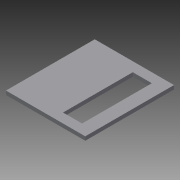
# Autodesk Inventor part: Step Down Regulator Adaptor
Saved by Autodesk Inventor 2015 (Build 190159000, 159)
## iProperties
Created: 2017-12-31
Part Number: Step Down Regulator Adaptor
Material: Generic
Document SubType Name: Modeling
Designer: Toby
Density: 1 g/cm^3
Appearance: Default
Author: Toby
Autodesk Inventor part; units mm, degrees
ref_plane "YZ Plane" through (0, 0, 0) normal (1, 0, 0) x (0, 1, 0)
ref_plane "XZ Plane" through (0, 0, 0) normal (0, 1, 0) x (-1, 0, 0)
ref_plane "XY Plane" through (0, 0, 0) normal (0, 0, 1) x (1, 0, 0)
sketch "Sketch1" plane through (0, 0, 0) normal (0, 0, 1) x (1, 0, 0)
  line L0 (-18.7121, 1.0985) -> (6.2879, 1.0985)
  line L1 (6.2879, 1.0985) -> (6.2879, -26.9015)
  line L2 (6.2879, -26.9015) -> (-18.7121, -26.9015)
  line L3 (-18.7121, -26.9015) -> (-18.7121, 1.0985)
  point P0 (0, 0)
  dimension "d0" = 25
  dimension "d1" = 28
  constraints: 8 end point, 2 parallel, 1 horizontal, 1 perpendicular
  measures "d0" distance of L0.start L0.end
  measures "d1" distance of L2.end L0.start
extrude "Extrusion1" add sketch "Sketch1" along normal blind 1.2
sketch "Sketch2" plane through (0, 0, 1.2) normal (0, 0, 1) x (1, 0, 0)
  line L0 (-3.7121, -1.9015) -> (2.2879, -1.9015)
  line L1 (2.2879, -1.9015) -> (2.2879, -23.9015)
  line L2 (2.2879, -23.9015) -> (-3.7121, -23.9015)
  line L3 (-3.7121, -23.9015) -> (-3.7121, -1.9015)
  line L4 (-18.7121, 1.0985) -> (-18.7121, -26.9015) projected
  line L5 (-18.7121, 1.0985) -> (6.2879, 1.0985) projected
  line L6 (6.2879, -26.9015) -> (-18.7121, -26.9015) projected
  point P0 (0, 0)
  dimension "d4" = 15
  dimension "d5" = 6
  dimension "d6" = 3
  dimension "d7" = 3
  constraints: 8 end point, 2 parallel, 1 horizontal, 1 perpendicular
  measures "d4" distance between parallel lines of L4 L3
  measures "d5" distance of L0.start L0.end
  measures "d6" distance between parallel lines of L5 L0
  measures "d7" distance between parallel lines of L6 L2
extrude "Extrusion2" cut sketch "Sketch2" against normal blind 1.2
body "Solid1"
